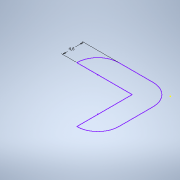
# Autodesk Inventor part: winkelTop
Saved by Autodesk Inventor 2020 (Build 240168000, 168)
## iProperties
Created: 2022-03-26
Part Number: winkelTop
Material: Kiefer
Document SubType Name: Modeling
Designer: Eric
Density: 0.570257 g/cm^3
Appearance: Gelbkiefer - massiv - natur - schwacher Glanz
Author: Eric
Autodesk Inventor part; units mm, degrees
ref_plane "YZ Plane" through (0, 0, 0) normal (1, 0, 0) x (0, 1, 0)
ref_plane "XZ Plane" through (0, 0, 0) normal (0, 1, 0) x (-1, 0, 0)
ref_plane "XY Plane" through (0, 0, 0) normal (0, 0, 1) x (1, 0, 0)
sketch "Skizze1" plane through (0, 0, 0) normal (0, 1, 0) x (-1, 0, 0)
  line L0 (-4.6, 12.6) -> (-4.6, 0)
  arc A0 (-4.6, 0) -> (0, -4.6) centre (0, 0) ccw
  line L1 (0, -4.6) -> (12.6, -4.6)
  arc A1 (12.6, -4.6) -> (17.2, 0) centre (12.6, 0) ccw
  line L2 (17.2, 0) -> (0, 0)
  line L3 (0, 0) -> (0, 17.2)
  arc A2 (0, 17.2) -> (-4.6, 12.6) centre (0, 12.6) ccw
  point P0 (0, 0)
  dimension "d0" = 4.6
  dimension "d1" = 21.8
  constraints: 8 end point, 6 point on circle, 4 tangent, 3 centre point, 3 perpendicular, 1 coincident, 1 line through centre, 1 parallel, 1 point on line, 1 vertical
  measures "d0" distance between parallel lines of L1 L2
  measures "d1" distance from line of L2.start L0
extrude "Extrusion1" add sketch "Skizze1" along normal blind 197.2
sketch "Skizze2" plane through (0, 0, -4.6) normal (0, 0, -1) x (-1, 0, 0)
  line L0 (-4.6, 0) -> (17.2, 21.8)
  line L1 (17.2, 0) -> (17.2, 197.2) projected
  line L2 (17.2, 0) -> (12.6, 0) projected
  line L3 (17.2, 21.8) -> (17.2, 0)
  line L4 (17.2, 0) -> (-4.6, 0)
  line L5 (17.2, 197.2) -> (-4.6, 197.2)
  line L6 (-4.6, 197.2) -> (17.2, 175.4)
  line L7 (17.2, 197.2) -> (17.2, 175.4)
  point P0 (0, 0)
  dimension "d4" = 45
  dimension "d7" = 45
  constraints: 12 end point, 2 point on line, 1 coincident, 1 collinear, 1 horizontal, 1 vertical
  measures "d4" angle of L0 L1
  measures "d7" angle of L1 L6
extrude "Extrusion2" cut sketch "Skizze2" against normal through all
sketch "Skizze3" plane through (4.6, 0, 0) normal (1, 0, 0) x (0, 0, -1)
  line L0 (4.6, 0) -> (-17.2, 21.8)
  line L1 (-17.2, 4.6) -> (-17.2, 192.6) projected
  line L2 (-17.2, 21.8) -> (-17.2, 0)
  line L3 (-17.2, 0) -> (4.6, 0)
  line L4 (-17.2, 175.4) -> (-17.2, 197.2)
  line L5 (-17.2, 197.2) -> (4.6, 197.2)
  line L6 (4.6, 197.2) -> (-17.2, 175.4)
  point P0 (0, 0)
  point P1 (4.6, 4.6)
  point P2 (-12.6, 197.2)
  dimension "d8" = 45
  dimension "d9" = 45
  constraints: 12 end point, 2 horizontal alignment, 2 point on line, 2 vertical, 2 vertical alignment, 1 horizontal, 1 perpendicular
  measures "d8" angle of L1 L0
  measures "d9" angle of L1 L6
extrude "Extrusion3" cut sketch "Skizze3" against normal through all
